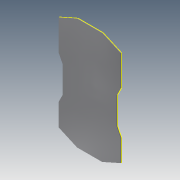
# Autodesk Inventor part: podvozek_sablona
Saved by Autodesk Inventor 2013 (Build 170138000, 138)
## iProperties
Created: 2012-08-22
Part Number: podvozek_sablona
Material: Generic
Document SubType Name: Modeling
Designer: idle-rug
Density: 1 g/cm^3
Author: idle-rug
Autodesk Inventor part; units mm, degrees
ref_plane "YZ Plane" through (0, 0, 0) normal (1, 0, 0) x (0, 1, 0)
ref_plane "XZ Plane" through (0, 0, 0) normal (0, 1, 0) x (-1, 0, 0)
ref_plane "XY Plane" through (0, 0, 0) normal (0, 0, 1) x (1, 0, 0)
sketch "Sketch1" plane through (0, 0, 0) normal (0, 1, 0) x (-1, 0, 0)
  line L0 (-75.5, -115.65) -> (-75.5, -62.65)
  line L1 (-65.5, -42.65) -> (-75.5, -62.65)
  line L2 (75.5, -115.65) -> (75.5, -62.65)
  line L3 (65.5, -42.65) -> (75.5, -62.65)
  line L4 (-75.5, 115.65) -> (-75.5, 42.15)
  line L5 (-65.5, 22.15) -> (-75.5, 42.15)
  line L6 (75.5, 115.65) -> (75.5, 42.15)
  line L7 (65.5, 22.15) -> (75.5, 42.15)
  line L8 (30.5, 135.65) -> (75.5, 115.65)
  line L9 (-30.5, 135.65) -> (-75.5, 115.65)
  line L10 (30.5, -135.65) -> (75.5, -115.65)
  line L11 (-30.5, -135.65) -> (-75.5, -115.65)
  line L12 (65.5, 22.15) -> (65.5, -42.65)
  line L13 (-65.5, -42.65) -> (-65.5, 22.15)
  line L14 (30.5, -135.65) -> (-30.5, -135.65)
  line L15 (30.5, 135.65) -> (-30.5, 135.65)
  constraints: 32 end point, 2 parallel, 1 perpendicular, 1 point on line
extrude "Extrusion1" add sketch "Sketch1" along normal blind 2
sketch "Sketch2" plane through (0, 2, 0) normal (0, 1, 0) x (1, 0, 0)
  circle A0 centre (-70.5, 110.65) radius 1.2
  circle A1 centre (-70.5, 67.65) radius 1.2
  circle A2 centre (70.5, 110.65) radius 1.2
  circle A3 centre (70.5, 67.65) radius 1.2
  circle A4 centre (0, 17.65) radius 1.2
  circle A5 centre (-60.5, 17.65) radius 1.2
  circle A6 centre (60.5, 17.65) radius 1.2
  circle A7 centre (-32.15, -17.15) radius 1.2
  circle A8 centre (32.15, -17.15) radius 1.2
  circle A9 centre (70.5, -42.15) radius 1.2
  circle A10 centre (70.5, -67.65) radius 1.2
  circle A11 centre (70.5, -110.65) radius 1.2
  circle A12 centre (-70.5, -67.65) radius 1.2
  circle A13 centre (-70.5, -110.65) radius 1.2
  circle A14 centre (-70.5, -42.15) radius 1.2
  circle A15 centre (0, -67.65) radius 1.2
  circle A16 centre (0, 110.65) radius 1.2
  circle A17 centre (-24.1, 67.65) radius 1.2
  circle A18 centre (24.1, 67.65) radius 1.2
  circle A19 centre (-24.1, -110.65) radius 1.2
  circle A20 centre (24.1, -110.65) radius 1.2
  circle A21 centre (-45.6, 89.15) radius 1.2
  circle A22 centre (45.6, 89.15) radius 1.2
  circle A23 centre (45.6, -89.15) radius 1.2
  circle A24 centre (-45.6, -89.15) radius 1.2
  line L0 (75.5, 62.65) -> (75.5, 115.65) projected
  line L1 (75.5, 115.65) -> (30.5, 135.65) projected
  line L2 (30.5, 135.65) -> (-30.5, 135.65) projected
  line L3 (-30.5, 135.65) -> (-75.5, 115.65) projected
  line L4 (-75.5, 115.65) -> (-75.5, 62.65) projected
  line L5 (-75.5, 62.65) -> (-65.5, 42.65) projected
  line L6 (-65.5, 42.65) -> (-65.5, -22.15) projected
  line L7 (-65.5, -22.15) -> (-75.5, -42.15) projected
  line L8 (-75.5, -42.15) -> (-75.5, -115.65) projected
  line L9 (-75.5, -115.65) -> (-30.5, -135.65) projected
  line L10 (-30.5, -135.65) -> (30.5, -135.65) projected
  line L11 (30.5, -135.65) -> (75.5, -115.65) projected
  line L12 (75.5, -115.65) -> (75.5, -42.15) projected
  line L13 (75.5, -42.15) -> (65.5, -22.15) projected
  line L14 (65.5, -22.15) -> (65.5, 42.65) projected
  line L15 (65.5, 42.65) -> (75.5, 62.65) projected
  constraints: 25 centre point
sketch "Sketch5" plane through (0, 2, 0) normal (0, 1, 0) x (1, 0, 0)
  line L0 (75.5, 62.65) -> (75.5, 115.65) projected
  line L1 (75.5, 115.65) -> (30.5, 135.65) projected
  line L2 (30.5, 135.65) -> (-30.5, 135.65) projected
  line L3 (-30.5, 135.65) -> (-75.5, 115.65) projected
  line L4 (-75.5, 115.65) -> (-75.5, 62.65) projected
  line L5 (-75.5, 62.65) -> (-65.5, 42.65) projected
  line L6 (-65.5, 42.65) -> (-65.5, -22.15) projected
  line L7 (-65.5, -22.15) -> (-75.5, -42.15) projected
  line L8 (-75.5, -42.15) -> (-75.5, -115.65) projected
  line L9 (-75.5, -115.65) -> (-30.5, -135.65) projected
  line L10 (-30.5, -135.65) -> (30.5, -135.65) projected
  line L11 (30.5, -135.65) -> (75.5, -115.65) projected
  line L12 (75.5, -115.65) -> (75.5, -42.15) projected
  line L13 (75.5, -42.15) -> (65.5, -22.15) projected
  line L14 (65.5, -22.15) -> (65.5, 42.65) projected
  line L15 (65.5, 42.65) -> (75.5, 62.65) projected
  point P0 (0, 0)
sketch "Sketch6" plane through (0, 2, 0) normal (0, 1, 0) x (1, 0, 0)
  line L0 (75.5, 62.65) -> (75.5, 115.65) projected
  line L1 (75.5, 115.65) -> (30.5, 135.65) projected
  line L2 (30.5, 135.65) -> (-30.5, 135.65) projected
  line L3 (-30.5, 135.65) -> (-75.5, 115.65) projected
  line L4 (-75.5, 115.65) -> (-75.5, 62.65) projected
  line L5 (-75.5, 62.65) -> (-65.5, 42.65) projected
  line L6 (-65.5, 42.65) -> (-65.5, -22.15) projected
  line L7 (-65.5, -22.15) -> (-75.5, -42.15) projected
  line L8 (-75.5, -42.15) -> (-75.5, -115.65) projected
  line L9 (-75.5, -115.65) -> (-30.5, -135.65) projected
  line L10 (-30.5, -135.65) -> (30.5, -135.65) projected
  line L11 (30.5, -135.65) -> (75.5, -115.65) projected
  line L12 (75.5, -115.65) -> (75.5, -42.15) projected
  line L13 (75.5, -42.15) -> (65.5, -22.15) projected
  line L14 (65.5, -22.15) -> (65.5, 42.65) projected
  line L15 (65.5, 42.65) -> (75.5, 62.65) projected
  point P0 (0, 0)
sketch "Sketch7" plane through (0, 2, 0) normal (0, 1, 0) x (1, 0, 0)
  line L0 (75.5, 62.65) -> (75.5, 115.65) projected
  line L1 (75.5, 115.65) -> (30.5, 135.65) projected
  line L2 (30.5, 135.65) -> (-30.5, 135.65) projected
  line L3 (-30.5, 135.65) -> (-75.5, 115.65) projected
  line L4 (-75.5, 115.65) -> (-75.5, 62.65) projected
  line L5 (-75.5, 62.65) -> (-65.5, 42.65) projected
  line L6 (-65.5, 42.65) -> (-65.5, -22.15) projected
  line L7 (-65.5, -22.15) -> (-75.5, -42.15) projected
  line L8 (-75.5, -42.15) -> (-75.5, -115.65) projected
  line L9 (-75.5, -115.65) -> (-30.5, -135.65) projected
  line L10 (-30.5, -135.65) -> (30.5, -135.65) projected
  line L11 (30.5, -135.65) -> (75.5, -115.65) projected
  line L12 (75.5, -115.65) -> (75.5, -42.15) projected
  line L13 (75.5, -42.15) -> (65.5, -22.15) projected
  line L14 (65.5, -22.15) -> (65.5, 42.65) projected
  line L15 (65.5, 42.65) -> (75.5, 62.65) projected
  point P0 (0, 0)
body "Solid1"
